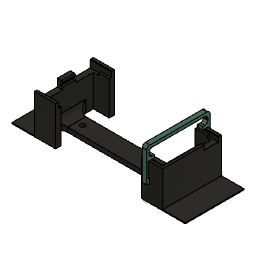
T-CAN485 holder v9 (Autodesk Fusion 360 design; units mm, degrees)
Autodesk Fusion 360 part; units mm, degrees
sketch "board" plane through (0, 0, 0) normal (0, 1, 0) x (1, 0, 0)
  line L0 (40.5, 17.5) -> (-40.5, 17.5)
  line L1 (-40.5, 17.5) -> (-40.5, -17.5)
  line L2 (-40.5, -17.5) -> (40.5, -17.5)
  line L3 (40.5, -17.5) -> (40.5, 17.5)
  line L4 (40.5, 17.5) -> (-40.5, -17.5) construction
  line L5 (-40.5, 17.5) -> (40.5, -17.5) construction
  line L6 (0, 0) -> (-107.5073, 0) construction
  line L7 (-40.5, 17.5) -> (-53.5, 17.5)
  line L8 (-53.5, 17.5) -> (-53.5, 4.3)
  line L9 (-53.5, 4.3) -> (-40.5, 4.3)
  line L10 (-40.5, 4.3) -> (-40.5, 17.5)
  line L11 (-40.5, -17.5) -> (-53.5, -17.5)
  line L12 (-53.5, -17.5) -> (-53.5, -4.3)
  line L13 (-53.5, -4.3) -> (-40.5, -4.3)
  line L14 (-40.5, -4.3) -> (-40.5, -17.5)
  line L15 (40.5, 17.5) -> (53.5, 17.5)
  line L16 (53.5, 17.5) -> (53.5, 8)
  line L17 (53.5, 8) -> (40.5, 8)
  line L18 (40.5, 8) -> (40.5, 17.5)
  line L19 (6.5, 17.5) -> (21.5, 17.5)
  line L20 (21.5, 17.5) -> (21.5, 37.5)
  line L21 (21.5, 37.5) -> (6.5, 37.5)
  line L22 (6.5, 37.5) -> (6.5, 17.5)
  point P0 (14, 17.5)
  dimension "d1" = 81
  dimension "d2" = 35
  dimension "d3" = 13
  dimension "d4" = 13.2
  dimension "d5" = 13
  dimension "d6" = 13.2
  dimension "d7" = 13
  dimension "d8" = 9.5
  dimension "d9" = 15
  dimension "d10" = 20
  dimension "d11" = 26.5
  constraint horizontal L0
  constraint perpendicular L0 L1
  constraint parallel L0 L2
  constraint parallel L1 L3
  constraint coincident L4 L6.start
  constraint coincident L5 L6.start
  constraint coincident L6.start origin
  constraint perpendicular L1 L6
  constraint horizontal L7
  constraint vertical L8
  constraint horizontal L9
  constraint vertical L10
  constraint horizontal L11
  constraint vertical L12
  constraint horizontal L13
  constraint vertical L14
  constraint horizontal L15
  constraint vertical L16
  constraint horizontal L17
  constraint vertical L18
  constraint horizontal L19
  constraint vertical L20
  constraint horizontal L21
  constraint vertical L22
  constraint coincident L0 L19.start
  constraint midpoint L19 P0
  measures "d1" distance of L1.end L2.end
  measures "d2" distance of L0.end L1.end
  measures "d3" distance of L0.end L7.end
  measures "d4" distance of L0.end L9.end
  measures "d5" distance of L1.end L11.end
  measures "d6" distance of L1.end L13.end
  measures "d7" distance of L0.start L15.end
  measures "d8" distance of L0.start L17.end
  measures "d9" distance of L19.start L19.end
  measures "d10" distance of L19.start L21.end
  measures "d11" distance of L0.start P0
extrude "Extrude1" add sketch "board" against normal blind 1.5 contours L0 L1 L2 L3 L10 L14 L18 L19 makes body 1
extrude "Extrude2" add sketch "board" along normal blind 11 from surface at -3 contours L3 L15 L16 L17 L18 | L0 L19 L20 L21 L22 | L1 L7 L8 L9 L10 | L1 L11 L12 L13 L14 bodies 1
ref_plane "WorkPlane1" through (0, -24, 0) normal (0, 1, 0) x (1, 0, 0)
sketch "base" plane through (0, -24, 0) normal (0, 1, 0) x (1, 0, 0)
  line L0 (-40.5, 17.5) -> (-40.5, 4.3)
  line L1 (-40.5, 4.3) -> (-40.5, -4.3)
  line L2 (-40.5, -4.3) -> (-40.5, -17.5)
  line L3 (-40.5, -17.5) -> (40.5, -17.5)
  line L4 (40.5, -17.5) -> (40.5, 8)
  line L5 (40.5, 8) -> (40.5, 17.5)
  line L6 (40.5, 17.5) -> (21.5, 17.5)
  line L7 (21.5, 17.5) -> (6.5, 17.5)
  line L8 (6.5, 17.5) -> (-40.5, 17.5)
  line L9 (53.5, 17.5) -> (53.5, 8)
  line L10 (53.5, 8) -> (40.5, 8)
  line L11 (40.5, 17.5) -> (53.5, 17.5)
  line L12 (40.5, 8) -> (40.5, -17.5)
  line L13 (-53.5, -17.5) -> (-53.5, -4.3)
  line L14 (-53.5, -4.3) -> (-40.5, -4.3)
  line L15 (-40.5, -17.5) -> (-53.5, -17.5)
  line L16 (21.5, 37.5) -> (6.5, 37.5)
  line L17 (21.5, 17.5) -> (21.5, 37.5)
  line L18 (6.5, 37.5) -> (6.5, 17.5)
  line L19 (21.5, 17.5) -> (40.5, 17.5)
  line L20 (-40.5, 17.5) -> (6.5, 17.5)
  line L21 (-40.5, 17.5) -> (-53.5, 17.5)
  line L22 (-53.5, 4.3) -> (-40.5, 4.3)
  line L23 (-53.5, 17.5) -> (-53.5, 4.3)
  line L24 (40.5, -17.5) -> (-40.5, -17.5)
  line L25 (-40.5, -4.3) -> (-40.5, 4.3)
  line L26 (28.5, 19.5) -> (42.5, 19.5)
  line L27 (42.5, 19.5) -> (42.5, -19.5)
  line L28 (42.5, -19.5) -> (28.5, -19.5)
  line L29 (28.5, -19.5) -> (28.5, 19.5)
  line L30 (40.5, -17.5) -> (40.5, 17.5)
  line L31 (-40.5, -17.5) -> (40.5, -17.5)
  line L32 (40.5, 17.5) -> (-40.5, 17.5)
  line L33 (0, -20) -> (0, -2.5)
  line L34 (-28.5, 19.5) -> (-42.5, 19.5)
  line L35 (-42.5, 19.5) -> (-42.5, -19.5)
  line L36 (-28.5, -19.5) -> (-28.5, 19.5)
  line L37 (-42.5, -19.5) -> (-28.5, -19.5)
  line L38 (28.5, 16) -> (39, 16)
  line L39 (39, 16) -> (39, -16)
  line L40 (39, -16) -> (28.5, -16)
  line L41 (28.5, -16) -> (28.5, 16)
  line L42 (40.5, 8) -> (40.5, 17.5)
  line L43 (-28.5, 16) -> (-39, 16)
  line L44 (-39, 16) -> (-39, -16)
  line L45 (-39, -16) -> (-28.5, -16)
  line L46 (39, -6) -> (-39, -6)
  line L47 (-39, -6) -> (-39, 6)
  line L48 (-39, 6) -> (39, 6)
  line L49 (39, 6) -> (39, -6)
  line L50 (39, -6) -> (-39, 6) construction
  line L51 (-39, -6) -> (39, 6) construction
  line L52 (0, 0) -> (42.5, 0) construction
  circle A0 centre (30, 0) radius 1.6
  circle A1 centre (-30, 0) radius 1.6
  dimension "d18" = 2
  dimension "d19" = 2
  dimension "d20" = 2
  dimension "d21" = 12
  dimension "d22" = 1.5
  dimension "d23" = 1.5
  dimension "d24" = 1.5
  dimension "d25" = 12
  dimension "d26" = 3.2
  dimension "d27" = 30
  constraint horizontal L26
  constraint vertical L27
  constraint horizontal L28
  constraint vertical L29
  constraint symmetric L26.start L33 L34.start
  constraint symmetric L26.end L33 L34.end
  constraint symmetric L27.end L33 L35.end
  constraint symmetric L28.end L33 L36.start
  constraint horizontal L38
  constraint vertical L39
  constraint horizontal L40
  constraint vertical L41
  constraint coincident L29 L38.start
  constraint symmetric L33 L38.start L43.start
  constraint symmetric L33 L38.end L43.end
  constraint symmetric L33 L39.end L44.end
  constraint symmetric L33 L40.end L45.end
  constraint horizontal L46
  constraint perpendicular L46 L47
  constraint parallel L46 L48
  constraint parallel L47 L49
  constraint coincident L50 L52.start
  constraint coincident L51 L52.start
  constraint coincident L52.start origin
  constraint midpoint L27 L52.end
  constraint coincident L52 A0.centre
  constraint symmetric L33 A0 A1
  constraint collinear L39 L49
  measures "d18" distance of L27 L30
  measures "d19" distance of L28 L31
  measures "d20" distance of L26 L32
  measures "d21" distance of L29 L30
  measures "d22" distance of L32 L38
  measures "d23" distance of L39 L42
  measures "d24" distance of L31 L40
  measures "d25" distance of L46.end L47.end
  measures "d26" diameter of A0
  measures "d27" distance of L33 A0.centre
extrude "Extrude3" add sketch "base" along normal blind 3 separate body contours L29 L36 L41 L46 L48 A0 A1 | L36 L44 L46 L47 L48 A1 | L29 L39 L41 L46 L48 L49 A0 makes body 2
extrude "Extrude4" add sketch "base" along normal up to surface (24 mm away) separate body contours L0 L1 L2 L3 L8 L20 L24 L25 L31 L32 L36 L43 L44 L45 L47 | L8 L20 L21 L32 L34 L35 L36 | L0 L21 L22 L35 | L1 L14 L22 L25 L35 | L2 L14 L15 L35 | L3 L15 L24 L31 L35 L36 L37 | L6 L11 L19 L26 L27 L29 L32 | L3 L4 L5 L6 L12 L19 L24 L29 L30 L31 L32 L38 L39 L40 L42 L49 | L5 L10 L11 L27 L30 L42 | L3 L4 L10 L12 L24 L27 L28 L29 L30 L31 makes body 3 at (42.5, -16, -6.5) makes body 4 at (-42.5, -16, -6.5)
combine "Combine1" operation add target body 3 tool bodies 2 4
combine "Combine2" operation cut target body 3 tool bodies 1 keep tools
sketch "can end latch" plane through (0, 0, -4.3) normal (0, 0, 1) x (1, 0, 0)
  line L0 (-53.5, -3) -> (-40.5, -3)
  line L1 (-40.5, -3) -> (-40.5, -1.5)
  line L2 (-40.5, -1.5) -> (-40.5, 0)
  line L3 (-40.5, 0) -> (-40.5, 8)
  line L4 (-40.5, 8) -> (-53.5, 8)
  line L5 (-53.5, 8) -> (-53.5, -3)
  line L6 (40.5, 0) -> (-40.5, 0)
  line L7 (-40.5, 0) -> (-40.5, 8)
  line L8 (-40.5, 8) -> (-53.5, 8)
  line L9 (-53.5, 8) -> (-53.5, -3)
  line L10 (-53.5, -3) -> (-40.5, -3)
  line L11 (-40.5, -3) -> (-40.5, -1.5)
  line L12 (-40.5, -1.5) -> (40.5, -1.5)
  line L13 (40.5, -1.5) -> (40.5, 0)
  line L14 (-28.5, 0) -> (-42.5, 0)
  line L15 (-42.5, 0) -> (-42.5, -24)
  line L16 (-42.5, -24) -> (-28.5, -24)
  line L17 (-28.5, -24) -> (-28.5, 0)
  line L18 (-42.5, 0) -> (-39, 0)
  line L19 (-39, 0) -> (-39, 2)
  line L20 (-39, 2) -> (-42.5, 2)
  line L21 (-42.5, 2) -> (-42.5, 0)
  dimension "d32" = 3.5
  dimension "d33" = 2
  constraint horizontal L18
  constraint vertical L19
  constraint horizontal L20
  constraint vertical L21
  constraint coincident L14.end L15.start
  measures "d32" distance of L14.end L18.end
  measures "d33" distance of L14.end L20.end
extrude "Extrude5" add sketch "can end latch" along normal up to surface (8.6 mm away) contours L3 L7 L14 L18 L20 L21 | L3 L6 L7 L14 L18 L19 L20 bodies 3
move_face "OffsetFaces1" offset -5 2 faces at (-40.5, -2, 8.7) (-40.5, -2.5, -13.1) on bodies 3
chamfer "Chamfer1" distance 0.7 angle 45 2 edges at (-39, 0, 0) (-39, 2, 0) on bodies 3
move_face "OffsetFaces2" offset -4 1 faces at (40.5, -2.5, -11.1667) on bodies 3
sketch "spacers" plane through (0, -24, 0) normal (0, -1, 0) x (1, 0, 0)
  circle A0 centre (-30, 0) radius 1.6
  circle A1 centre (30, 0) radius 1.6
  line L0 (39, -16) -> (28.5, -16)
  line L1 (28.5, -16) -> (28.5, -19.5)
  line L2 (28.5, -19.5) -> (42.5, -19.5)
  line L3 (42.5, -19.5) -> (42.5, 19.5)
  line L4 (42.5, 19.5) -> (28.5, 19.5)
  line L5 (28.5, 19.5) -> (28.5, 16)
  line L6 (28.5, 16) -> (39, 16)
  line L7 (39, 16) -> (39, 6)
  line L8 (39, 6) -> (-39, 6)
  line L9 (-39, 6) -> (-39, 16)
  line L10 (-39, 16) -> (-28.5, 16)
  line L11 (-28.5, 16) -> (-28.5, 19.5)
  line L12 (-28.5, 19.5) -> (-42.5, 19.5)
  line L13 (-42.5, 19.5) -> (-42.5, -19.5)
  line L14 (-42.5, -19.5) -> (-28.5, -19.5)
  line L15 (-28.5, -19.5) -> (-28.5, -16)
  line L16 (-28.5, -16) -> (-39, -16)
  line L17 (-39, -16) -> (-39, -6)
  line L18 (-39, -6) -> (39, -6)
  line L19 (39, -6) -> (39, -16)
  line L20 (57.5, -19.5) -> (-57.5, -19.5)
  line L21 (-57.5, -19.5) -> (-57.5, 19.5)
  line L22 (-57.5, 19.5) -> (57.5, 19.5)
  line L23 (57.5, 19.5) -> (57.5, -19.5)
  line L24 (57.5, -19.5) -> (-57.5, 19.5) construction
  line L25 (-57.5, -19.5) -> (57.5, 19.5) construction
  dimension "d56" = 115
  constraint horizontal L20
  constraint perpendicular L20 L21
  constraint parallel L20 L22
  constraint parallel L21 L23
  constraint coincident L24 origin
  constraint coincident L25 origin
  measures "d56" distance of L21.end L22.end
extrude "Extrude9" add sketch "spacers" against normal blind 0.6 contours L3 L20 L22 L23 | L13 L20 L21 L22 bodies 3
fillet "Fillet1" radius 5 6 edges at (-39, -21, 0) (39, -21, 0) (39, -22.5, 6) (39, -22.5, -6) (-39, -22.5, 6) (-39, -22.5, -6) on bodies 3
sketch "Sketch7" plane through (28.5, 0, 0) normal (-1, 0, 0) x (0, 0, 1)
  line L0 (17.5, 0) -> (17.5, -1.5)
  line L1 (17.5, -1.5) -> (16, -1.5)
  line L2 (16, -1.5) -> (16, -24)
  line L3 (16, -24) -> (19.5, -24)
  line L4 (19.5, -24) -> (19.5, 0)
  line L5 (19.5, 0) -> (17.5, 0)
  line L6 (-17.5, -1.5) -> (-17.5, 0)
  line L7 (-17.5, 0) -> (-19.5, 0)
  line L8 (-19.5, 0) -> (-19.5, -24)
  line L9 (-19.5, -24) -> (-16, -24)
  line L10 (-16, -24) -> (-16, -1.5)
  line L11 (-16, -1.5) -> (-17.5, -1.5)
  line L12 (19.5, 0) -> (16, 0)
  line L13 (16, 0) -> (16, 2)
  line L14 (16, 2) -> (19.5, 2)
  line L15 (19.5, 2) -> (19.5, 0)
  line L16 (19.5, 2) -> (21, 2)
  line L17 (21, 2) -> (21, -13)
  line L18 (21, -13) -> (19.5, -13)
  line L19 (19.5, -13) -> (19.5, 2)
  line L20 (19.5, -13) -> (16.5, -13)
  line L21 (16.5, -13) -> (16.5, -10)
  line L22 (16.5, -10) -> (19.5, -10)
  line L23 (19.5, -10) -> (19.5, -13)
  line L24 (0, 0) -> (0, 22.9783) construction
  line L25 (21, 2) -> (19.5, 2)
  line L26 (19.5, 2) -> (19.5, 7)
  line L27 (19.5, 7) -> (21, 7)
  line L28 (21, 7) -> (21, 2)
  line L29 (21, 7) -> (0, 7)
  line L30 (0, 7) -> (0, 9)
  line L31 (0, 9) -> (21, 9)
  line L32 (21, 9) -> (21, 7)
  line L33 (19.5, -10) -> (19.8, -10)
  line L34 (19.8, -10) -> (19.8, 0)
  line L35 (19.8, 0) -> (19.5, 0)
  dimension "d61" = 2
  dimension "d62" = 1.5
  dimension "d63" = 15
  dimension "d64" = 3
  dimension "d65" = 3
  dimension "d66" = 5
  dimension "d67" = 2
  dimension "d81" = 0.3
  constraint horizontal L12
  constraint vertical L13
  constraint horizontal L14
  constraint vertical L15
  constraint coincident L4.end L5.start
  constraint collinear L2 L13
  constraint horizontal L16
  constraint vertical L17
  constraint horizontal L18
  constraint vertical L19
  constraint horizontal L20
  constraint vertical L21
  constraint horizontal L22
  constraint vertical L23
  constraint coincident L24.start origin
  constraint vertical L24
  constraint horizontal L25
  constraint vertical L26
  constraint horizontal L27
  constraint vertical L28
  constraint horizontal L29
  constraint vertical L30
  constraint horizontal L31
  constraint vertical L32
  constraint collinear L19 L26
  constraint perpendicular L4 L33
  constraint perpendicular L12 L34
  constraint perpendicular L4 L35
  measures "d61" distance of L4.end L14.end
  measures "d62" distance of L14.end L16.end
  measures "d63" distance of L14.end L18.end
  measures "d64" distance of L18.end L20.end
  measures "d65" distance of L18.end L22.end
  measures "d66" distance of L16.end L27.end
  measures "d67" distance of L27.end L31.end
  measures "d81" distance of L22.end L33.end
extrude "Extrude10" add sketch "Sketch7" against normal blind 3 from surface at -2 separate body contours L5 L12 L13 L14 L15 L19 | L4 L15 L16 L17 L18 L19 L23 L25 L33 L34 L35 | L4 L19 L20 L21 L22 L23 | L16 L25 L26 L27 L28 L29 | L27 L29 L30 L31 L32 makes body 5
sketch "Sketch8" plane through (0, 0, 19.5) normal (0, 0, 1) x (1, 0, 0)
  line L0 (42.5, 0) -> (28.5, 0)
  line L1 (28.5, 0) -> (28.5, -24)
  line L2 (28.5, -24) -> (57.5, -24)
  line L3 (57.5, -24) -> (57.5, -23.4)
  line L4 (57.5, -23.4) -> (42.5, -23.4)
  line L5 (42.5, -23.4) -> (42.5, 0)
  line L6 (30.5, -13) -> (30.5, -10)
  line L7 (30.5, -10) -> (33.5, -10)
  line L8 (33.5, -10) -> (33.5, -13)
  line L9 (33.5, -13) -> (30.5, -13)
  line L10 (30.2, -13.3) -> (30.2, -9.7)
  line L11 (30.2, -9.7) -> (33.8, -9.7)
  line L12 (33.8, -9.7) -> (33.8, -13.3)
  line L13 (33.8, -13.3) -> (30.2, -13.3)
  dimension "d71" = -0.3
extrude "Extrude11" cut sketch "Sketch8" against normal blind 100 contours L6 L7 L8 L9 | L10 L11 L12 L13 bodies 3
fillet "Fillet2" radius 2 3 edges at (32, 2, 19.5) (32, 7, 19.5) (32, 9, 21) on bodies 5
chamfer "Chamfer3" distance 0.5 angle 45 1 faces at (32.5, -12, 16.5) on bodies 5
mirror "Mirror2" about plane through (0, 0, 0) normal (0, 0, 1) of bodies 5 merged
move_face "OffsetFaces3" offset 2 2 faces at (-37.8333, 0, 18.1667) (-37.8333, 0, -18.1667) on bodies 3
chamfer "Chamfer4" distance 0.3 angle 45 5 edges at (-35.5, 2, -17.5) (-35.5, 2, 17.5) (40.5, 0, 4.75) (35.5, 0, -17.5) (34.5, 0, 17.5) on bodies 3
chamfer "Chamfer5" distance 0.3 angle 45 2 edges at (30.5, -5, 19.8) (33.5, -5, 19.8) on bodies 5
hidden bodies 1
named bodies: "board", "t-can485 holder", "t-can485 clip"
